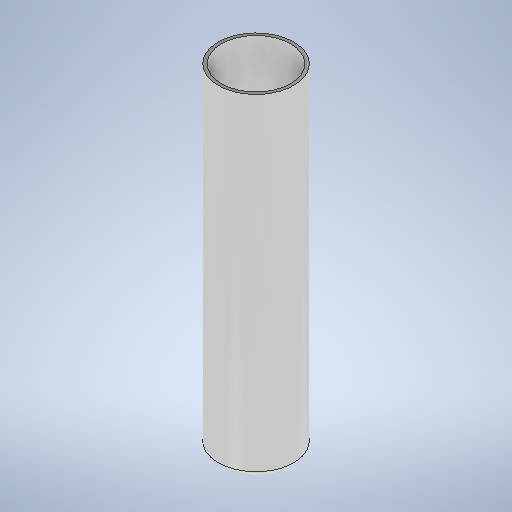
# Autodesk Inventor part: Jack_obudowa
Saved by Autodesk Inventor 2025 (Build 290162000, 162)
## iProperties
Created: 2026-04-03
Part Number: Jack_obudowa
Material: Ogólny
Document SubType Name: Modeling
Designer: zzapa
Density: 1 g/cm^3
Appearance: Chrom — polerowany
Author: zzapa
Autodesk Inventor part; units mm, degrees
ref_plane "YZ Plane" through (0, 0, 0) normal (1, 0, 0) x (0, 1, 0)
ref_plane "XZ Plane" through (0, 0, 0) normal (0, 1, 0) x (-1, 0, 0)
sketch "Szkic1" plane through (0, 0, 0) normal (0, 1, 0) x (-1, 0, 0)
  circle A0 centre (0, 0) radius 6
  dimension "d0" = 12
  constraints: 1 centre point, 1 coincident
  measures "d0" diameter of A0
extrude "Wyciągnięcie proste1" add sketch "Szkic1" along normal blind 53
sketch "Szkic2" plane through (0, 53, 0) normal (0, 1, 0) x (1, 0, 0)
  point P0 (0, 0)
  point P1 (0, 0)
  constraints: 1 coincident
ref_plane "Płaszczyzna konstrukcyjna1" through (0, 2, 0) normal (0, -1, 0) x (1, 0, 0)
hole "Otwór1" at (0, 53, 0) direction (0, -1, 0) diameter 11 depth 51
sketch "Szkic3" plane through (0, 0, 0) normal (0, -1, 0) x (1, 0, 0)
  point P0 (0, 0)
  point P1 (0, 0)
  constraints: 1 coincident
hole "Otwór2" at (0, 0, 0) direction (0, 1, 0) diameter 7 end through all
fillet "Zaokrąglenie1" radius 1 1 edges at (6, 0, 0)
